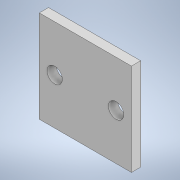
# Autodesk Inventor part: space_plate
Saved by Autodesk Inventor 2022 (Build 260153000, 153)
## iProperties
Created: 2022-01-31
Part Number: space_plate
Material: Generic
Document SubType Name: Modeling
Designer: Martijn
Density: 1 g/cm^3
Appearance: Default
Author: Martijn
Autodesk Inventor part; units mm, degrees
ref_plane "YZ Plane" through (0, 0, 0) normal (1, 0, 0) x (0, 1, 0)
ref_plane "XZ Plane" through (0, 0, 0) normal (0, 1, 0) x (-1, 0, 0)
ref_plane "XY Plane" through (0, 0, 0) normal (0, 0, 1) x (1, 0, 0)
sketch "Sketch1" plane through (0, 0, 0) normal (0, 0, 1) x (1, 0, 0)
  point P0 (0, 0)
sketch "Sketch2" plane through (0, 0, 0) normal (0, 0, 1) x (1, 0, 0)
  line L0 (0, 0) -> (30, 0)
  line L1 (30, 0) -> (30, 30)
  line L2 (30, 30) -> (0, 30)
  line L3 (0, 30) -> (0, 0)
  dimension "d0" = 30
  dimension "d1" = 30
  constraints: 8 end point, 2 parallel, 1 horizontal, 1 perpendicular
  measures "d0" distance between parallel lines of L0 L2
  measures "d1" distance between parallel lines of L3 L1
extrude "Extrusion1" add sketch "Sketch2" along normal blind 3
sketch "Sketch3" plane through (0, 0, 3) normal (0, 0, 1) x (1, 0, 0)
  circle A0 centre (5, 15) radius 2.5
  circle A1 centre (25, 15) radius 2.5
  line L0 (0, 0) -> (30, 0) projected
  line L1 (30, 0) -> (30, 30) projected
  line L2 (0, 30) -> (0, 0) projected
  dimension "d4" = 15
  dimension "d5" = 15
  dimension "d6" = 5
  dimension "d7" = 5
  dimension "d8" = 5
  constraints: 2 centre point, 1 equal radius
  measures "d4" distance from line of L0 A0.centre
  measures "d5" distance from line of L0 A1.centre
  measures "d6" distance from line of L1 A1.centre
  measures "d7" distance from line of L2 A0.centre
  measures "d8" diameter of A0
extrude "Extrusion2" cut sketch "Sketch3" against normal blind 3
body "Solid1"
